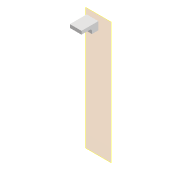
# Autodesk Inventor part: Mounting Bracket Bottom
Saved by Autodesk Inventor 2020 (Build 240168000, 168)
## iProperties
Created: 2019-11-16
Part Number: Mounting Bracket Bottom
Material: Generic
Document SubType Name: Modeling
Designer: ball
Density: 1 g/cm^3
Appearance: Default
Author: ball
Autodesk Inventor part; units mm, degrees
ref_plane "YZ Plane" through (0, 0, 0) normal (1, 0, 0) x (0, 1, 0)
ref_plane "XZ Plane" through (0, 0, 0) normal (0, 1, 0) x (-1, 0, 0)
ref_plane "XY Plane" through (0, 0, 0) normal (0, 0, 1) x (1, 0, 0)
ref_plane "Work Plane1" through (0, 0, 0) normal (0, 0, 1) x (1, 0, 0)
sketch "Sketch1" plane through (0, 0, 0) normal (0, 0, 1) x (1, 0, 0)
  line L0 (17.75, 85) -> (-18.004, 85) construction
  circle A0 centre (-7.75, 70) radius 1.7 construction
  line L1 (-9.375, 72.8146) -> (-6.125, 72.8146) construction
  line L2 (-18.004, 85) -> (-18.004, -85) construction
  line L3 (-3.25, 73.1895) -> (-3.25, 76.1105) construction
  line L4 (-11, 70) -> (-9.375, 72.8146) construction
  line L5 (3.2502, 74.65) -> (3.2502, 77.444) construction
  line L6 (3.2502, 77.825) -> (3.2502, 81) construction
  line L7 (-0.127, 85) -> (-18.004, 85)
  line L8 (-18.004, 85) -> (-18.004, 72.8146)
  line L9 (-18.004, 72.8146) -> (-0.127, 72.8146)
  line L10 (-0.127, 72.8146) -> (-0.127, 85)
  circle A1 centre (-7.75, 76.8764) radius 1.7
  point P0 (0, 0)
  dimension "d0" = 3.4
  dimension "d1" = 12.1854
  dimension "d3" = 17.877
  dimension "d6" = 4.0618
  constraints: 8 end point, 2 parallel, 1 centre point, 1 horizontal, 1 midpoint, 1 perpendicular, 1 point on line
  measures "d0" diameter of A1
  measures "d1" distance between parallel lines of L7 L9
  measures "d3" distance of L0.end L7.start
  measures "d6" vertical distance of L1.start A1.centre
extrude "Leg" add sketch "Sketch1" along normal blind 10
sketch "Sketch2" plane through (0, 0, 10) normal (0, 0, 1) x (1, 0, 0)
  line L0 (-0.127, 72.8146) -> (-0.127, 85) projected
  line L1 (-18.004, 85) -> (-18.004, 72.8146) projected
  line L2 (-18.004, 85) -> (-18.004, 80.9625)
  line L3 (-0.127, 80.9625) -> (-0.127, 85)
  line L4 (-0.127, 85) -> (-18.004, 85)
  line L5 (-18.004, 85) -> (-18.004, 79.92)
  line L6 (-18.004, 79.92) -> (-0.127, 79.92)
  line L7 (-0.127, 79.92) -> (-0.127, 85)
  point P0 (0, 0)
  dimension "d7" = 5.08
  constraints: 12 end point, 3 parallel, 2 point on line, 1 horizontal, 1 perpendicular
  measures "d7" distance of L5.end L4.end
extrude "Extrusion2" add sketch "Sketch2" along normal blind 16
fillet "Fillet1" radius 3.175 1 edges at (-9.0655, 79.92, 10)
equation "\"d6\" = 0.333333 * d1"
body "Solid1"
